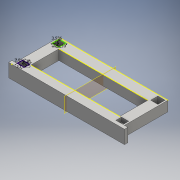
# Autodesk Inventor part: Front Facing Beam Support
Saved by Autodesk Inventor 2016 (Build 200138000, 138)
## iProperties
Created: 2016-04-05
Part Number: Front Facing Beam Support
Material: Generic
Document SubType Name: Modeling
Designer: Kenneth Daniel
Density: 1 g/cm^3
Appearance: Default
Author: Kenneth Daniel
Autodesk Inventor part; units mm, degrees
ref_plane "YZ Plane" through (0, 0, 0) normal (1, 0, 0) x (0, 1, 0)
ref_plane "XZ Plane" through (0, 0, 0) normal (0, 1, 0) x (-1, 0, 0)
ref_plane "XY Plane" through (0, 0, 0) normal (0, 0, 1) x (1, 0, 0)
sketch "Sketch1" plane through (0, 0, 0) normal (0, 0, 1) x (1, 0, 0)
  line L0 (0, 0) -> (0, 70)
  line L1 (0, 70) -> (163, 70)
  line L2 (163, 70) -> (163, 0)
  line L3 (163, 0) -> (0, 0)
  line L4 (0, 70) -> (15, 70)
  line L5 (15, 55) -> (15, 13)
  line L6 (0, 70) -> (0, 55)
  line L7 (15, 55) -> (148, 55)
  line L8 (163, 70) -> (148, 70)
  line L9 (148, 55) -> (148, 13)
  line L10 (163, 0) -> (163, 13)
  line L11 (148, 13) -> (15, 13)
  dimension "d0" = 70
  dimension "d1" = 163
  dimension "d2" = 15
  dimension "d3" = 15
  dimension "d4" = 15
  dimension "d5" = 13
  constraints: 24 end point, 5 perpendicular, 4 point on line, 2 parallel, 1 vertical
  measures "d0" distance of L0.start L0.end
  measures "d1" distance of L0.end L1.end
  measures "d2" distance of L0.end L4.end
  measures "d3" distance of L0.end L6.end
  measures "d4" distance of L1.end L8.end
  measures "d5" distance of L2.end L10.end
extrude "Extrusion1" add sketch "Sketch1" along normal blind 15
sketch "Sketch2" plane through (0, 0, 0) normal (0, 0, -1) x (-1, 0, 0)
  line L0 (-163, 0) -> (-163, 70) projected
  line L1 (-163, 0) -> (-163, 5)
  line L2 (-163, 5) -> (0, 5)
  line L3 (0, 0) -> (-163, 0) projected
  line L4 (-163, 0) -> (0, 0)
  line L5 (-163, 0) -> (0, 0)
  line L6 (0, 0) -> (0, 5)
  line L7 (0, 5) -> (-163, 5)
  line L8 (-163, 5) -> (-163, 0)
  dimension "d8" = 5
  constraints: 14 end point, 3 equal length, 2 perpendicular, 1 horizontal, 1 point on line
  measures "d8" distance of L0.start L1.end
extrude "Extrusion2" add sketch "Sketch2" along normal blind 5
sketch "Sketch3" plane through (163, 0, 15) normal (1, 0, 0) x (0, 0, -1)
  line L0 (20, 5) -> (20, 0) projected
  line L1 (0, 0) -> (20, 0)
  line L2 (20, 0) -> (20, 5)
  line L3 (20, 5) -> (0, 5)
  line L4 (0, 5) -> (0, 0)
  point P0 (15, 0)
  constraints: 8 end point, 2 parallel, 1 horizontal, 1 perpendicular
extrude "Extrusion3" add sketch "Sketch3" along normal blind 5
ref_plane "Work Plane1" through (81.5, 70, 15) normal (1, 0, 0) x (0, 0, -1)
mirror "Mirror1" about plane through (81.5, 70, 15) normal (1, 0, 0) of "Extrusion3"
sketch "Sketch4" plane through (0, 0, 15) normal (0, 0, 1) x (1, 0, 0)
  line L0 (163, 70) -> (0, 70) projected
  line L1 (15, 55) -> (148, 55) projected
  line L2 (0, 70) -> (2.5003, 67.4997) construction
  line L3 (2.5003, 67.4997) -> (2.5003, 57.4997)
  line L4 (2.5003, 57.4997) -> (12.5003, 57.4997)
  line L5 (12.5003, 57.4997) -> (12.5003, 67.4997)
  line L6 (12.5003, 67.4997) -> (2.5003, 67.4997)
  line L7 (148, 13) -> (15, 13) projected
  line L8 (15, 13) -> (12.5, 13) construction
  line L9 (12.5, 13) -> (2.5, 13)
  line L10 (2.5, 13) -> (2.5, 5.5)
  line L11 (2.5, 5.5) -> (12.5, 5.5)
  line L12 (12.5, 5.5) -> (12.5, 13)
  line L13 (2.1, 13.4) -> (12.9, 13.4)
  line L14 (12.9, 13.4) -> (12.9, 5.1)
  line L15 (12.9, 5.1) -> (2.1, 5.1)
  line L16 (2.1, 5.1) -> (2.1, 13.4)
  line L17 (12.9003, 57.0997) -> (2.1003, 57.0997)
  line L18 (2.1003, 57.0997) -> (2.1003, 67.8997)
  line L19 (2.1003, 67.8997) -> (12.9003, 67.8997)
  line L20 (12.9003, 67.8997) -> (12.9003, 57.0997)
  point P0 (0, 0)
  dimension "d13" = 3.536
  dimension "d14" = 10
  dimension "d15" = 10
  dimension "d16" = 10
  dimension "d17" = 2.5
  dimension "d18" = 10
  dimension "d19" = 7.5
  dimension "d20" = 10
  dimension "d22" = 0.4
  dimension "d23" = 0.4
  constraints: 36 end point, 6 perpendicular, 1 horizontal, 1 point on line, 1 vertical, 6 other
  measures "d13" distance of L0.end L2.end
  measures "d14" distance of L2.end L3.end
  measures "d15" distance of L3.end L4.end
  measures "d16" distance of L4.end L5.end
  measures "d17" distance of L7.end L8.end
  measures "d18" distance of L8.end L9.end
  measures "d19" distance of L9.end L10.end
  measures "d20" distance of L10.end L11.end
  measures "d22" distance between parallel lines of L9 L13
  measures "d23" distance between parallel lines of L4 L17
extrude "Extrusion4" cut sketch "Sketch4" against normal blind 6.7 contours L12 L11 L10 L9 | L13 L14 L15 L16
extrude "Extrusion5" cut sketch "Sketch4" against normal blind 14.2 contours L6 L5 L4 L3 | L17 L18 L19 L20
mirror "Mirror2" about plane through (81.5, 70, 15) normal (1, 0, 0) of "Extrusion4", "Extrusion5"
body "Solid1"
